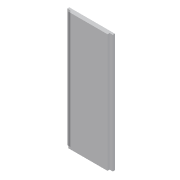
# Autodesk Inventor part: Lid_MaintenanceCover
Saved by Autodesk Inventor 2016 (Build 200138000, 138)
## iProperties
Created: 2016-07-04
Part Number: Lid_MaintenanceCover
Material: Polycarbonat, klar
Document SubType Name: Modeling
Designer: Gero Hofmann
Density: 1.2 g/cm^3
Appearance: Polycarbonat - klar
Author: Gero Hofmann
Autodesk Inventor part; units mm, degrees
ref_plane "YZ Plane" through (0, 0, 0) normal (1, 0, 0) x (0, 1, 0)
ref_plane "XZ Plane" through (0, 0, 0) normal (0, 1, 0) x (-1, 0, 0)
ref_plane "XY Plane" through (0, 0, 0) normal (0, 0, 1) x (1, 0, 0)
sketch "Skizze1" plane through (0, 0, 0) normal (0, 0, 1) x (1, 0, 0)
  line L0 (73, -6) -> (-73, -6)
  line L1 (-73, -6) -> (-73, 6)
  line L2 (-73, 6) -> (73, 6)
  line L3 (73, 6) -> (73, -6)
  line L4 (73, -6) -> (-73, 6) construction
  line L5 (-73, -6) -> (73, 6) construction
  point P0 (0, 0)
  dimension "d0" = 146
  dimension "d1" = 12
  constraints: 12 end point, 2 midpoint, 2 parallel, 1 horizontal, 1 perpendicular
  measures "d0" distance of L1.end L2.end
  measures "d1" distance of L0.end L1.end
extrude "Extrusion1" add sketch "Skizze1" along normal blind 289
sketch "Skizze2" plane through (0, 0, 0) normal (0, 0, -1) x (-1, 0, 0)
  line L0 (-73, -6) -> (-64, -6)
  line L1 (-64, -6) -> (-64, 0)
  line L2 (-64, 0) -> (-73, 0)
  line L3 (-73, 0) -> (-73, -6)
  line L4 (73, -6) -> (64, -6)
  line L5 (64, -6) -> (64, 0)
  line L6 (64, 0) -> (73, 0)
  line L7 (73, 0) -> (73, -6)
  point P0 (0, 0)
  dimension "d4" = 6
  dimension "d5" = 128
  dimension "d6" = 64
  constraints: 16 end point, 5 parallel, 2 horizontal, 2 perpendicular
  measures "d4" distance of L1.end L0.end
  measures "d5" distance between parallel lines of L5 L1
  measures "d6" distance from line of point (0, 0) L1
extrude "Extrusion2" cut sketch "Skizze2" against normal through all
equation "\"d6\" = 0.5 * d5"
